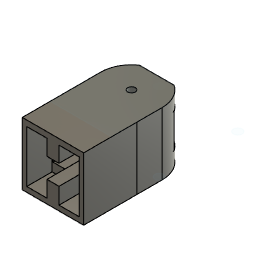
EndCap__FreeWheel (Autodesk Fusion 360 design; units mm, degrees)
Autodesk Fusion 360 part; units mm, degrees
(part 1 of 2)
sketch "Sketch1" plane through (0, 0, 0) normal (1, 0, 0) x (0, 0, -1)
  line L0 (0, 0) -> (-20, 0)
  line L1 (-20, 0) -> (-20, 20)
  line L2 (-20, 20) -> (0, 20)
  line L3 (0, 20) -> (0, 0)
  line L4 (-6.34, 6.34) -> (-13.66, 6.34)
  line L5 (-13.66, 6.34) -> (-13.66, 13.66)
  line L6 (-13.66, 13.66) -> (-6.34, 13.66)
  line L7 (-6.34, 13.66) -> (-6.34, 6.34)
  line L8 (-6.34, 6.34) -> (-13.66, 13.66) construction
  line L9 (-13.66, 6.34) -> (-6.34, 13.66) construction
  line L10 (-20, 20) -> (-20, 18.5)
  line L11 (-20, 18.5) -> (-18.5, 18.5)
  line L12 (-18.5, 18.5) -> (-1.5, 18.5)
  line L13 (-1.5, 18.5) -> (-1.5, 1.5)
  line L14 (-1.5, 1.5) -> (-18.5, 1.5)
  line L15 (-18.5, 1.5) -> (-18.5, 18.5)
  line L16 (-20, 0) -> (-20, 7.37)
  line L17 (-20, 7.37) -> (0, 7.37)
  line L18 (0, 7.37) -> (0, 12.63)
  line L19 (0, 12.63) -> (-20, 12.63)
  line L20 (-20, 12.63) -> (-20, 7.37)
  line L21 (-20, 0) -> (-12.63, 0)
  line L22 (-12.63, 0) -> (-7.37, 0)
  line L23 (-7.37, 0) -> (-7.37, 20.1614)
  line L24 (-7.37, 20.1614) -> (-12.63, 20.1614)
  line L25 (-12.63, 20.1614) -> (-12.63, 0)
  line L26 (-18.5, 18.5) -> (-1.5, 1.5)
  line L27 (-10, 10) -> (-9.4697, 10.5303)
  line L28 (-9.4697, 10.5303) -> (-17.4393, 18.5)
  line L29 (-9.4697, 10.5303) -> (1.8011, 10.5303) construction
  line L30 (-9.4697, 10.5303) -> (-1.5, 2.5607)
  line L31 (-10, 10) -> (-10.5303, 9.4697)
  line L32 (-10.5303, 9.4697) -> (-18.5, 17.4393)
  line L33 (-10.5303, 9.4697) -> (-2.5607, 1.5)
  line L34 (-10, 10) -> (-9.4697, 9.4697)
  line L35 (-9.4697, 9.4697) -> (-1.5, 17.4393)
  line L36 (-9.4697, 9.4697) -> (-17.4393, 1.5)
  line L37 (-10, 10) -> (-10.5303, 10.5303)
  line L38 (-10.5303, 10.5303) -> (-2.5607, 18.5)
  line L39 (-10.5303, 10.5303) -> (-18.5, 2.5607)
  line L40 (-10, 18.5) -> (-4.005, 18.5)
  line L41 (-4.005, 18.5) -> (-15.995, 18.5)
  line L42 (-15.995, 18.5) -> (-15.995, 17.0557)
  line L43 (-15.995, 17.0557) -> (-4.005, 17.0557)
  line L44 (-4.005, 17.0557) -> (-4.005, 18.5)
  line L45 (-15.995, 1.5) -> (-4.005, 1.5)
  line L46 (-4.005, 1.5) -> (-4.005, 2.9443)
  line L47 (-4.005, 2.9443) -> (-15.995, 2.9443)
  line L48 (-15.995, 2.9443) -> (-15.995, 1.5)
  line L49 (-18.5, 10) -> (-18.5, 4.005)
  line L50 (-18.5, 4.005) -> (-17.0557, 4.005)
  line L51 (-17.0557, 4.005) -> (-17.0557, 15.995)
  line L52 (-17.0557, 15.995) -> (-18.5, 15.995)
  line L53 (-18.5, 15.995) -> (-18.5, 4.005)
  line L54 (-1.5, 10) -> (-1.5, 4.005)
  line L55 (-1.5, 4.005) -> (-2.9443, 4.005)
  line L56 (-2.9443, 4.005) -> (-2.9443, 15.995)
  line L57 (-2.9443, 15.995) -> (-1.5, 15.995)
  line L58 (-1.5, 15.995) -> (-1.5, 4.005)
  point P0 (-10, 10)
  dimension "d1" = 20
  dimension "d2" = 20
  dimension "d3" = 7.32
  dimension "d4" = 7.32
  dimension "d5" = 1.5
  dimension "d6" = 1.5
  dimension "d7" = 17
  dimension "d8" = 17
  dimension "d9" = 7.37
  dimension "d10" = 5.26
  dimension "d11" = 7.37
  dimension "d12" = 5.26
  dimension "d13" = 0.75
  dimension "d14" = 135
  dimension "d15" = 45
  dimension "d16" = 0.75
  dimension "d17" = 0.75
  dimension "d18" = 0.75
  dimension "d19" = 5.995
  dimension "d20" = 11.99
  dimension "d21" = 11.99
  dimension "d22" = 5.995
  dimension "d23" = 11.99
  dimension "d24" = 5.995
  dimension "d25" = 11.99
  constraint horizontal L0
  constraint vertical L1
  constraint horizontal L2
  constraint vertical L3
  constraint coincident L0.start L3.end
  constraint perpendicular L4 L5
  constraint parallel L4 L6
  constraint parallel L5 L7
  constraint horizontal L4
  constraint coincident L8 P0
  constraint coincident L9 P0
  constraint perpendicular L2 L10
  constraint perpendicular L1 L11
  constraint horizontal L12
  constraint vertical L13
  constraint horizontal L14
  constraint vertical L15
  constraint perpendicular L0 L16
  constraint horizontal L17
  constraint vertical L18
  constraint horizontal L19
  constraint vertical L20
  constraint perpendicular L1 L21
  constraint horizontal L22
  constraint vertical L23
  constraint horizontal L24
  constraint vertical L25
  constraint coincident P0 L27.start
  constraint perpendicular L26 L27
  constraint horizontal L29
  constraint coincident L12 L28.end
  constraint coincident L13 L30.end
  constraint perpendicular L26 L31
  constraint coincident L15 L32.end
  constraint perpendicular L31 L32
  constraint coincident L14 L33.end
  constraint perpendicular L31 L33
  constraint perpendicular L31 L34
  constraint coincident L13 L35.end
  constraint perpendicular L30 L35
  constraint coincident L14 L36.end
  constraint perpendicular L34 L36
  constraint perpendicular L31 L37
  constraint coincident L12 L38.end
  constraint perpendicular L37 L38
  constraint coincident L15 L39.end
  constraint perpendicular L37 L39
  constraint midpoint L12 L40.start
  constraint perpendicular L23 L40
  constraint horizontal L41
  constraint vertical L42
  constraint horizontal L43
  constraint vertical L44
  constraint coincident L28 L42.end
  constraint horizontal L45
  constraint vertical L46
  constraint horizontal L47
  constraint vertical L48
  constraint coincident L33 L46.end
  constraint coincident L14 L45.start
  constraint vertical L49
  constraint midpoint L15 L49.start
  constraint horizontal L50
  constraint vertical L51
  constraint horizontal L52
  constraint vertical L53
  constraint coincident L32 L51.end
  constraint vertical L54
  constraint midpoint L13 L54.start
  constraint horizontal L55
  constraint vertical L56
  constraint horizontal L57
  constraint vertical L58
  constraint coincident L35 L56.end
  measures "d1" distance of L0.start L0.end
  measures "d2" distance of L0.start L2.end
  measures "d3" distance of L5.end L6.end
  measures "d4" distance of L4.end L5.end L0.start
  measures "d5" distance of L1.end L10.end
  measures "d6" distance of L10.end L11.end
  measures "d7" distance of L11.end L14.end
  measures "d8" distance of L11.end L12.end
  measures "d9" distance of L0.end L16.end
  measures "d10" distance of L16.end L19.end
  measures "d11" distance of L0.end L21.end
  measures "d12" distance of L21.end L22.end
  measures "d13" distance of P0 L27.end
  measures "d14" angle of L28 L29
  measures "d15" angle of L29 L30
  measures "d16" distance of P0 L31.end
  measures "d17" distance of P0 L34.end
  measures "d18" distance of P0 L37.end
  measures "d19" distance of L40.start L40.end
  measures "d20" distance of L40.end L41.end
  measures "d21" distance of L45.start L45.end
  measures "d22" distance of L49.start L49.end
  measures "d23" distance of L49.end L52.end
  measures "d24" distance of L54.start L54.end
  measures "d25" distance of L54.end L57.end
extrude "Extrude1" add sketch "Sketch1" along normal blind 10 contours L0 L3 L13 L14 L17 L23 L45 L54 L58 | L0 L1 L14 L15 L16 L17 L21 L25 L45 L49 L53 | L2 L3 L12 L13 L19 L23 L40 L41 L58 | L14 L33 L46 | L13 L30 L55 | L14 L36 L48 | L4 L14 L23 L26 L33 | L13 L35 L57 | L7 L13 L17 L26 L30 | L1 L11 L15 L19 L53 | L4 L5 L14 L15 L17 L25 L36 L39 | L4 L23 L26 | L4 L17 L23 L33 | L4 L17 L33 L36 | L1 L2 L10 L11 L12 L25 L41 | L6 L7 L12 L13 L19 L23 L35 L38 | L7 L17 L23 L30 | L7 L17 L26 | L7 L23 L30 L35 | L15 L39 L50 | L4 L17 L25 L36 | L4 L5 L17 L25 | L23 L26 L30 L35 | L17 L26 L33 L36 | L17 L33 L36 | L12 L38 L44 | L6 L7 L19 L23 | L7 L19 L23 L35 | L23 L30 L35 | L5 L15 L19 L26 L32 | L6 L12 L25 L26 L28 | L17 L25 L32 L33 L36 L39 | L5 L17 L25 L39 | L26 L31 L33 L34 L36 | L26 L27 L30 L34 L35 | L19 L23 L28 L30 L35 L38 | L6 L19 L23 L38 | L5 L19 L26 | L6 L25 L26 | L5 L25 L32 L39 | L25 L32 L39 | L26 L31 L32 L37 L39 | L26 L27 L28 L37 L38 | L6 L19 L28 L38 | L19 L28 L38 | L5 L19 L25 L32 | L6 L19 L25 L28 | L25 L26 L32 L39 | L19 L26 L28 L38 makes body 1
sketch "Sketch2" plane through (10, 0, 0) normal (1, 0, 0) x (0, 0, -1)
  line L0 (-6.3093, 12.63) -> (-2.9443, 15.995)
  line L1 (-2.9443, 15.995) -> (-1.5, 15.995)
  line L2 (-1.5, 15.995) -> (-1.5, 12.63)
  line L3 (-1.5, 12.63) -> (0, 12.63)
  line L4 (0, 12.63) -> (0, 20)
  line L5 (0, 20) -> (-7.37, 20)
  line L6 (-7.37, 20) -> (-7.37, 18.5)
  line L7 (-7.37, 18.5) -> (-4.005, 18.5)
  line L8 (-4.005, 18.5) -> (-4.005, 17.0557)
  line L9 (-4.005, 17.0557) -> (-7.37, 13.6907)
  line L10 (-7.37, 13.6907) -> (-7.37, 13.66)
  line L11 (-7.37, 13.66) -> (-12.63, 13.66)
  line L12 (-12.63, 13.66) -> (-12.63, 13.6907)
  line L13 (-12.63, 13.6907) -> (-17.4393, 18.5)
  line L14 (-17.4393, 18.5) -> (-12.63, 18.5)
  line L15 (-12.63, 18.5) -> (-12.63, 20)
  line L16 (-12.63, 20) -> (-20, 20)
  line L17 (-20, 20) -> (-20, 12.63)
  line L18 (-20, 12.63) -> (-18.5, 12.63)
  line L19 (-18.5, 12.63) -> (-18.5, 17.4393)
  line L20 (-18.5, 17.4393) -> (-13.6907, 12.63)
  line L21 (-13.6907, 12.63) -> (-13.66, 12.63)
  line L22 (-13.66, 12.63) -> (-13.66, 7.37)
  line L23 (-13.66, 7.37) -> (-13.6907, 7.37)
  line L24 (-13.6907, 7.37) -> (-17.0557, 4.005)
  line L25 (-17.0557, 4.005) -> (-18.5, 4.005)
  line L26 (-18.5, 4.005) -> (-18.5, 7.37)
  line L27 (-18.5, 7.37) -> (-20, 7.37)
  line L28 (-20, 7.37) -> (-20, 0)
  line L29 (-20, 0) -> (-12.63, 0)
  line L30 (-12.63, 0) -> (-12.63, 1.5)
  line L31 (-12.63, 1.5) -> (-15.995, 1.5)
  line L32 (-15.995, 1.5) -> (-15.995, 2.9443)
  line L33 (-15.995, 2.9443) -> (-12.63, 6.3093)
  line L34 (-12.63, 6.3093) -> (-12.63, 6.34)
  line L35 (-12.63, 6.34) -> (-7.37, 6.34)
  line L36 (-7.37, 6.34) -> (-7.37, 6.3093)
  line L37 (-7.37, 6.3093) -> (-4.005, 2.9443)
  line L38 (-4.005, 2.9443) -> (-4.005, 1.5)
  line L39 (-4.005, 1.5) -> (-7.37, 1.5)
  line L40 (-7.37, 1.5) -> (-7.37, 0)
  line L41 (-7.37, 0) -> (0, 0)
  line L42 (0, 0) -> (0, 7.37)
  line L43 (0, 7.37) -> (-1.5, 7.37)
  line L44 (-1.5, 7.37) -> (-1.5, 4.005)
  line L45 (-1.5, 4.005) -> (-2.9443, 4.005)
  line L46 (-2.9443, 4.005) -> (-6.3093, 7.37)
  line L47 (-6.3093, 7.37) -> (-6.34, 7.37)
  line L48 (-6.34, 7.37) -> (-6.34, 12.63)
  line L49 (-6.34, 12.63) -> (-6.3093, 12.63)
  line L50 (-6.34, 10) -> (-10, 10)
  circle A0 centre (-10, 10) radius 2.095
  dimension "d28" = 4.19
  constraint midpoint L48 L50.start
  constraint perpendicular L48 L50
  constraint coincident L50.end A0.centre
  measures "d28" diameter of A0
extrude "Extrude2" cut sketch "Sketch2" against normal blind 10 contours A0 bodies 1
fillet "Fillet1" radius 1.5 4 edges at (5, 0, 0) (5, 0, 20) (5, 20, 0) (5, 20, 20) on bodies 1
sketch "Sketch3" plane through (10, 0, 0) normal (1, 0, 0) x (0, 0, -1)
  arc A0 (-18.5, 20) -> (-20, 18.5) centre (-18.5, 18.5) ccw
  line L0 (-20, 18.5) -> (-20, 12.63)
  line L1 (-20, 12.63) -> (-18.5, 12.63)
  line L2 (-18.5, 12.63) -> (-18.5, 17.4393)
  line L3 (-18.5, 17.4393) -> (-13.6907, 12.63)
  line L4 (-13.6907, 12.63) -> (-13.66, 12.63)
  line L5 (-13.66, 12.63) -> (-13.66, 7.37)
  line L6 (-13.66, 7.37) -> (-13.6907, 7.37)
  line L7 (-13.6907, 7.37) -> (-17.0557, 4.005)
  line L8 (-17.0557, 4.005) -> (-18.5, 4.005)
  line L9 (-18.5, 4.005) -> (-18.5, 7.37)
  line L10 (-18.5, 7.37) -> (-20, 7.37)
  line L11 (-20, 7.37) -> (-20, 1.5)
  arc A1 (-20, 1.5) -> (-18.5, 0) centre (-18.5, 1.5) ccw
  line L12 (-18.5, 0) -> (-12.63, 0)
  line L13 (-12.63, 0) -> (-12.63, 1.5)
  line L14 (-12.63, 1.5) -> (-15.995, 1.5)
  line L15 (-15.995, 1.5) -> (-15.995, 2.9443)
  line L16 (-15.995, 2.9443) -> (-12.63, 6.3093)
  line L17 (-12.63, 6.3093) -> (-12.63, 6.34)
  line L18 (-12.63, 6.34) -> (-7.37, 6.34)
  line L19 (-7.37, 6.34) -> (-7.37, 6.3093)
  line L20 (-7.37, 6.3093) -> (-4.005, 2.9443)
  line L21 (-4.005, 2.9443) -> (-4.005, 1.5)
  line L22 (-4.005, 1.5) -> (-7.37, 1.5)
  line L23 (-7.37, 1.5) -> (-7.37, 0)
  line L24 (-7.37, 0) -> (-1.5, 0)
  arc A2 (-1.5, 0) -> (0, 1.5) centre (-1.5, 1.5) ccw
  line L25 (0, 1.5) -> (0, 7.37)
  line L26 (0, 7.37) -> (-1.5, 7.37)
  line L27 (-1.5, 7.37) -> (-1.5, 4.005)
  line L28 (-1.5, 4.005) -> (-2.9443, 4.005)
  line L29 (-2.9443, 4.005) -> (-6.3093, 7.37)
  line L30 (-6.3093, 7.37) -> (-6.34, 7.37)
  line L31 (-6.34, 7.37) -> (-6.34, 12.63)
  line L32 (-6.34, 12.63) -> (-6.3093, 12.63)
  line L33 (-6.3093, 12.63) -> (-2.9443, 15.995)
  line L34 (-2.9443, 15.995) -> (-1.5, 15.995)
  line L35 (-1.5, 15.995) -> (-1.5, 12.63)
  line L36 (-1.5, 12.63) -> (0, 12.63)
  line L37 (0, 12.63) -> (0, 18.5)
  arc A3 (0, 18.5) -> (-1.5, 20) centre (-1.5, 18.5) ccw
  line L38 (-1.5, 20) -> (-7.37, 20)
  line L39 (-7.37, 20) -> (-7.37, 18.5)
  line L40 (-7.37, 18.5) -> (-4.005, 18.5)
  line L41 (-4.005, 18.5) -> (-4.005, 17.0557)
  line L42 (-4.005, 17.0557) -> (-7.37, 13.6907)
  line L43 (-7.37, 13.6907) -> (-7.37, 13.66)
  line L44 (-7.37, 13.66) -> (-12.63, 13.66)
  line L45 (-12.63, 13.66) -> (-12.63, 13.6907)
  line L46 (-12.63, 13.6907) -> (-17.4393, 18.5)
  line L47 (-17.4393, 18.5) -> (-12.63, 18.5)
  line L48 (-12.63, 18.5) -> (-12.63, 20)
  line L49 (-12.63, 20) -> (-18.5, 20)
  circle A4 centre (-10, 10) radius 2.095
  line L50 (-4.005, 17.0557) -> (-15.995, 17.0557)
  line L51 (-17.0557, 4.005) -> (-17.0557, 15.995)
  line L52 (-17.0557, 15.995) -> (-18.5, 15.995)
  line L53 (-15.995, 17.0557) -> (-15.995, 18.5)
  constraint coincident L41.end L42.start
  constraint coincident L46 L50.end
  constraint perpendicular L41 L50
  constraint coincident L7.end L8.start
  constraint coincident L3 L51.end
  constraint perpendicular L8 L51
  constraint coincident L2 L52.end
  constraint perpendicular L2 L52
  constraint coincident L47 L53.end
  constraint perpendicular L47 L53
extrude "Extrude3" add sketch "Sketch3" against normal blind 10 contours L46 L47 L53 | L2 L3 L52 bodies 1
sketch "Sketch4" plane through (0, 0, 0) normal (0, 1, 0) x (1, 0, 0)
  line L0 (25, 0) -> (67, 0)
  line L1 (67, 0) -> (67, -42)
  line L2 (67, -42) -> (25, -42)
  line L3 (25, -42) -> (25, 0)
  line L4 (46, 0) -> (46, -21)
  line L5 (61.5, -36.5) -> (61.5, -5.5)
  line L6 (61.5, -5.5) -> (30.5, -36.5) construction
  line L7 (30.5, -5.5) -> (61.5, -36.5) construction
  circle A0 centre (30.5, -5.5) radius 1.75
  circle A1 centre (61.5, -5.5) radius 1.75
  circle A2 centre (30.5, -36.5) radius 1.75
  circle A3 centre (61.5, -36.5) radius 1.75
  point P0 (46, -21)
  dimension "d34" = 42
  dimension "d35" = 42
  dimension "d36" = 21
  dimension "d37" = 31
  dimension "d38" = 31
  dimension "d39" = 3.5
  dimension "d40" = 3.5
  dimension "d41" = 3.5
  dimension "d42" = 3.5
  constraint horizontal L0
  constraint vertical L1
  constraint horizontal L2
  constraint vertical L3
  constraint midpoint L0 L4.start
  constraint perpendicular L0 L4
  constraint coincident L6 P0
  constraint coincident L7 P0
  constraint coincident P0 L4.end
  constraint coincident L7.start A0.centre
  constraint coincident L5.end L6.start
  constraint coincident L6.end A2.centre
  constraint coincident L5.start L7.end
  measures "d34" distance of L0.start L2.end
  measures "d35" distance of L0.start L0.end
  measures "d36" distance of L4.start P0
  measures "d37" distance of L6.end L5.start
  measures "d38" distance of L7.start L6.end
  measures "d39" diameter of A0
  measures "d40" diameter of A1
  measures "d41" diameter of A2
  measures "d42" diameter of A3
extrude "Extrude4" add sketch "Sketch4" along normal blind 5 separate body makes body 2
sketch "Sketch5" plane through (25, 0, 0) normal (-1, 0, 0) x (0, 0, 1)
  line L0 (0, 0) -> (42, 0)
  line L1 (42, 0) -> (42, 5)
  line L2 (42, 5) -> (0, 5)
  line L3 (0, 5) -> (0, 0)
  line L4 (42, 0) -> (31, 0)
  line L5 (31, 0) -> (11, 0)
  line L6 (11, 0) -> (11, 20)
  line L7 (11, 20) -> (31, 20)
  line L8 (31, 20) -> (31, 0)
  line L9 (31, 0) -> (31, 1.5)
  line L10 (31, 1.5) -> (29.5, 1.5)
  line L11 (29.5, 1.5) -> (12.5, 1.5)
  line L12 (12.5, 1.5) -> (12.5, 18.5)
  line L13 (12.5, 18.5) -> (29.5, 18.5)
  line L14 (29.5, 18.5) -> (29.5, 1.5)
  line L15 (21, 1.5) -> (23.5, 1.5)
  line L16 (23.5, 1.5) -> (18.5, 1.5)
  line L17 (18.5, 1.5) -> (18.5, 0)
  line L18 (18.5, 0) -> (23.5, 0)
  line L19 (23.5, 0) -> (23.5, 1.5)
  line L20 (11, 10) -> (21, 10)
  line L21 (21, 10) -> (21.5303, 10.5303)
  line L22 (21, 10) -> (21.5303, 9.4697)
  line L23 (21, 10) -> (21.75, 10) construction
  line L24 (21.5303, 10.5303) -> (13.5607, 18.5)
  line L25 (21.5303, 10.5303) -> (29.5, 2.5607)
  line L26 (21.5303, 9.4697) -> (29.5, 17.4393)
  line L27 (21.5303, 9.4697) -> (13.5607, 1.5)
  line L28 (21, 10) -> (20.4697, 9.4697)
  line L29 (20.4697, 9.4697) -> (12.5, 17.4393)
  line L30 (21, 8.9393) -> (28.4393, 1.5)
  line L31 (21, 10) -> (20.4697, 10.5303)
  line L32 (20.4697, 10.5303) -> (12.5, 2.5607)
  line L33 (20.4697, 10.5303) -> (28.4393, 18.5)
  line L34 (24.66, 6.34) -> (17.34, 6.34)
  line L35 (17.34, 6.34) -> (17.34, 13.66)
  line L36 (17.34, 13.66) -> (24.66, 13.66)
  line L37 (24.66, 13.66) -> (24.66, 6.34)
  line L38 (24.66, 6.34) -> (17.34, 13.66) construction
  line L39 (17.34, 6.34) -> (24.66, 13.66) construction
  line L40 (21, 1.5) -> (26.75, 1.5)
  line L41 (26.75, 1.5) -> (15.25, 1.5)
  line L42 (15.25, 1.5) -> (15.25, 3.1893)
  line L43 (15.25, 3.1893) -> (26.75, 3.1893)
  line L44 (26.75, 3.1893) -> (26.75, 1.5)
  line L45 (15.25, 18.5) -> (26.75, 18.5)
  line L46 (26.75, 18.5) -> (26.75, 16.8107)
  line L47 (26.75, 16.8107) -> (15.25, 16.8107)
  line L48 (15.25, 16.8107) -> (15.25, 18.5)
  point P0 (21, 10)
  dimension "d45" = 20
  dimension "d46" = 20
  dimension "d47" = 1.5
  dimension "d48" = 1.5
  dimension "d49" = 2.5
  dimension "d50" = 5
  dimension "d51" = 1.5
  dimension "d53" = 0.75
  dimension "d54" = 45
  dimension "d55" = 0.75
  dimension "d56" = 0.75
  dimension "d57" = 7.32
  dimension "d58" = 7.32
  dimension "d59" = 5.75
  dimension "d60" = 11.5
  constraint coincident L0.end L1.start
  constraint coincident L0 L4.end
  constraint horizontal L5
  constraint vertical L6
  constraint horizontal L7
  constraint vertical L8
  constraint perpendicular L4 L9
  constraint perpendicular L8 L10
  constraint horizontal L11
  constraint vertical L12
  constraint horizontal L13
  constraint vertical L14
  constraint midpoint L11 L15.start
  constraint parallel L11 L15
  constraint horizontal L16
  constraint vertical L17
  constraint horizontal L18
  constraint vertical L19
  constraint midpoint L6 L20.start
  constraint perpendicular L14 L20
  constraint horizontal L23
  constraint perpendicular L21 L22
  constraint coincident L13 L24.end
  constraint perpendicular L21 L24
  constraint coincident L14 L25.end
  constraint perpendicular L21 L25
  constraint coincident L14 L26.end
  constraint perpendicular L25 L26
  constraint coincident L11 L27.end
  constraint perpendicular L22 L27
  constraint perpendicular L22 L28
  constraint coincident L12 L29.end
  constraint perpendicular L27 L29
  constraint coincident L27 L30.start
  constraint coincident L11 L30.end
  constraint perpendicular L27 L30
  constraint perpendicular L28 L31
  constraint coincident L12 L32.end
  constraint perpendicular L31 L32
  constraint coincident L13 L33.end
  constraint perpendicular L31 L33
  constraint perpendicular L34 L35
  constraint parallel L34 L36
  constraint parallel L35 L37
  constraint horizontal L34
  constraint coincident L38 P0
  constraint coincident L39 P0
  constraint coincident P0 L20.end
  constraint parallel L11 L40
  constraint horizontal L41
  constraint vertical L42
  constraint horizontal L43
  constraint vertical L44
  constraint coincident L27 L42.end
  constraint horizontal L45
  constraint vertical L46
  constraint horizontal L47
  constraint vertical L48
  constraint coincident L33 L46.end
  constraint coincident L13 L45.start
  measures "d45" distance of L4.end L7.end
  measures "d46" distance of L4.end L5.end
  measures "d47" distance of L4.end L9.end
  measures "d48" distance of L9.end L10.end
  measures "d49" distance of L15.start L15.end
  measures "d50" distance of L15.end L16.end
  measures "d51" distance of L15.end L18.end
  measures "d53" distance of P0 L21.end
  measures "d54" angle of L22 L23
  measures "d55" distance of P0 L22.end
  measures "d56" distance of P0 L31.end
  measures "d57" distance of L34.end L35.end
  measures "d58" distance of L35.end L36.end
  measures "d59" distance of L15.start L40.end
  measures "d60" distance of L40.end L41.end
extrude "Extrude5" add sketch "Sketch5" along normal blind 5 contours L11 L15 L16 L40 L41 L42 L43 L44 | L2 L27 L30 L43 | L2 L27 L30 L34 | L13 L45 L46 L47 L48 | L24 L33 L36 L47 bodies 2 makes body 3 at (23.3333, 18.5, 19.0833)
sketch "Sketch6" plane through (25, 0, 0) normal (-1, 0, 0) x (0, 0, 1)
  line L0 (15.25, 3.1893) -> (17.0607, 5)
  line L1 (17.0607, 5) -> (0, 5)
  line L2 (0, 5) -> (0, 0)
  line L3 (0, 0) -> (42, 0)
  line L4 (42, 0) -> (42, 5)
  line L5 (42, 5) -> (24.9393, 5)
  line L6 (24.9393, 5) -> (26.75, 3.1893)
  line L7 (26.75, 3.1893) -> (26.75, 1.5)
  line L8 (26.75, 1.5) -> (15.25, 1.5)
  line L9 (15.25, 1.5) -> (15.25, 3.1893)
  line L10 (42, 0) -> (31, 0)
  line L11 (31, 0) -> (11, 0)
  line L12 (11, 0) -> (11, 20)
  line L13 (11, 20) -> (31, 20)
  line L14 (31, 20) -> (31, 0)
  line L15 (24.9393, 5) -> (17.0603, 5)
  line L16 (17.0603, 5) -> (17.0603, 18.4957)
  line L17 (17.0603, 18.4957) -> (24.9393, 18.4957)
  line L18 (24.9393, 18.4957) -> (24.9393, 5)
  dimension "d63" = 20
  dimension "d64" = 20
  dimension "d65" = 7.879
  constraint coincident L3.end L4.start
  constraint coincident L3 L10.end
  constraint horizontal L11
  constraint vertical L12
  constraint horizontal L13
  constraint vertical L14
  constraint horizontal L15
  constraint vertical L16
  constraint horizontal L17
  constraint vertical L18
  constraint coincident L5.end L6.start
  measures "d63" distance of L10.end L11.end
  measures "d64" distance of L10.end L13.end
  measures "d65" distance of L5.end L15.end
extrude "Extrude6" add sketch "Sketch6" against normal blind 9 contours L15 L16 L17 L18 bodies 2 3
sketch "Sketch7" plane through (25, 0, 0) normal (-1, 0, 0) x (0, 0, 1)
  line L0 (18.4007, 13.66) -> (17.0603, 15.0003)
  line L1 (17.0603, 15.0003) -> (17.0603, 5)
  line L2 (17.0603, 5) -> (0, 5)
  line L3 (0, 5) -> (0, 0)
  line L4 (0, 0) -> (42, 0)
  line L5 (42, 0) -> (42, 5)
  line L6 (42, 5) -> (24.9393, 5)
  line L7 (24.9393, 5) -> (26.75, 3.1893)
  line L8 (26.75, 3.1893) -> (26.75, 1.5)
  line L9 (26.75, 1.5) -> (15.25, 1.5)
  line L10 (15.25, 1.5) -> (15.25, 3.1893)
  line L11 (15.25, 3.1893) -> (18.4007, 6.34)
  line L12 (18.4007, 6.34) -> (23.5993, 6.34)
  line L13 (23.5993, 6.34) -> (24.9393, 5)
  line L14 (24.9393, 5) -> (24.9393, 15)
  line L15 (24.9393, 15) -> (23.5993, 13.66)
  line L16 (23.5993, 13.66) -> (18.4007, 13.66)
  line L17 (21, 0) -> (23.5, 0)
  line L18 (23.5, 0) -> (18.5, 0)
  line L19 (18.5, 0) -> (18.5, 1.5)
  line L20 (18.5, 1.5) -> (23.5, 1.5)
  line L21 (23.5, 1.5) -> (23.5, 0)
  dimension "d68" = 2.5
  dimension "d69" = 5
  dimension "d70" = 1.5
  constraint midpoint L4 L17.start
  constraint parallel L4 L17
  constraint horizontal L18
  constraint vertical L19
  constraint horizontal L20
  constraint vertical L21
  measures "d68" distance of L17.start L17.end
  measures "d69" distance of L17.end L18.end
  measures "d70" distance of L17.end L20.end
extrude "Extrude7" add sketch "Sketch7" along normal blind 5 contours L4 L9 L17 L18 L19 L20 L21 bodies 2
sketch "Sketch8" plane through (34, 0, 0) normal (1, 0, 0) x (0, 0, -1)
  line L0 (-17.0603, 18.4957) -> (-24.9393, 18.4957)
  line L1 (-24.9393, 18.4957) -> (-24.9393, 5)
  line L2 (-24.9393, 5) -> (-17.0603, 5)
  line L3 (-17.0603, 5) -> (-17.0603, 18.4957)
  line L4 (-17.0603, 5) -> (-20.9998, 5)
  line L5 (-20.9998, 5) -> (-20.9998, 10)
  circle A0 centre (-20.9998, 10) radius 2.25
  dimension "d73" = 4.5
  constraint coincident L2.end L3.start
  constraint midpoint L2 L4.end
  constraint perpendicular L4 L5
  constraint coincident L5.end A0.centre
  measures "d73" diameter of A0
extrude "Extrude8" cut sketch "Sketch8" against normal blind 19 contours A0 bodies 2
sketch "Sketch9" plane through (20, 0, 0) normal (-1, 0, 0) x (0, 0, 1)
  line L0 (23.5993, 6.34) -> (18.4007, 6.34)
  line L1 (18.4007, 6.34) -> (15.25, 3.1893)
  line L2 (15.25, 3.1893) -> (15.25, 1.5)
  line L3 (15.25, 1.5) -> (18.5, 1.5)
  line L4 (18.5, 1.5) -> (18.5, 0)
  line L5 (18.5, 0) -> (23.5, 0)
  line L6 (23.5, 0) -> (23.5, 1.5)
  line L7 (23.5, 1.5) -> (26.75, 1.5)
  line L8 (26.75, 1.5) -> (26.75, 3.1893)
  line L9 (26.75, 3.1893) -> (23.5993, 6.34)
  line L10 (18.5, 1.5) -> (16.0303, 3.9697)
  line L11 (23.5, 1.5) -> (25.9697, 3.9697)
  constraint coincident L3.end L4.start
  constraint coincident L1 L10.end
  constraint perpendicular L1 L10
  constraint coincident L6.end L7.start
  constraint coincident L9 L11.end
  constraint perpendicular L9 L11
extrude "Extrude9" cut sketch "Sketch9" against normal blind 5 contours L7 L8 L9 L11 | L1 L2 L3 L10 bodies 2
sketch "Sketch10" plane through (0, 0, 0) normal (0, -1, 0) x (1, 0, 0)
  circle A0 centre (30.5, 5.5) radius 1.75
  circle A1 centre (30.5, 36.5) radius 1.75
  circle A2 centre (61.5, 5.5) radius 1.75
  circle A3 centre (61.5, 36.5) radius 1.75
  line L0 (67, 42) -> (25, 42)
  line L1 (25, 42) -> (25, 23.5)
  line L2 (25, 23.5) -> (20, 23.5)
  line L3 (20, 23.5) -> (20, 18.5)
  line L4 (20, 18.5) -> (25, 18.5)
  line L5 (25, 18.5) -> (25, 0)
  line L6 (25, 0) -> (67, 0)
  line L7 (67, 0) -> (67, 42)
  line L8 (46, 0) -> (46, 20)
  circle A4 centre (46, 20) radius 8.625
  dimension "d78" = 17.25
  constraint midpoint L6 L8.start
  constraint perpendicular L6 L8
  constraint coincident L8.end A4.centre
  measures "d78" diameter of A4
sketch "Sketch11" plane through (0, 0, 0) normal (0, -1, 0) x (1, 0, 0)
  circle A0 centre (30.5, 5.5) radius 1.75
  circle A1 centre (30.5, 36.5) radius 1.75
  circle A2 centre (61.5, 5.5) radius 1.75
  circle A3 centre (61.5, 36.5) radius 1.75
  line L0 (67, 42) -> (25, 42)
  line L1 (25, 42) -> (25, 23.5)
  line L2 (25, 23.5) -> (20, 23.5)
  line L3 (20, 23.5) -> (20, 18.5)
  line L4 (20, 18.5) -> (25, 18.5)
  line L5 (25, 18.5) -> (25, 0)
  line L6 (25, 0) -> (67, 0)
  line L7 (67, 0) -> (67, 42)
  circle A4 centre (46, 20) radius 12
  dimension "d81" = 24
  measures "d81" diameter of A4
extrude "Extrude12" add 2 faces at (20, 4.7267, 21.8333) (20, 16.8867, 21.8664) along direction (-1, 0, 0) blind 5 on bodies 2 bodies 2
sketch "Sketch12" plane through (0, 18.5, 0) normal (0, 1, 0) x (-1, 0, 0)
  line L0 (-25, 26.75) -> (-25, 15.25)
  line L1 (-25, 15.25) -> (-15, 15.25)
  line L2 (-15, 15.25) -> (-15, 26.75)
  line L3 (-15, 26.75) -> (-25, 26.75)
  line L4 (-15, 21) -> (-20, 21)
  circle A0 centre (-20, 21) radius 1.25
  dimension "d86" = 2.5
  constraint midpoint L2 L4.start
  constraint perpendicular L0 L4
  constraint coincident L4.end A0.centre
  measures "d86" diameter of A0
extrude "Extrude13" cut sketch "Sketch12" against normal blind 21 contours A0 bodies 2
sketch "Sketch13" plane through (0, 0, 0) normal (0, -1, 0) x (1, 0, 0)
  circle A0 centre (20, 21) radius 1.25
  circle A1 centre (30.5, 5.5) radius 1.75
  circle A2 centre (30.5, 36.5) radius 1.75
  circle A3 centre (61.5, 5.5) radius 1.75
  circle A4 centre (61.5, 36.5) radius 1.75
  line L0 (67, 42) -> (25, 42)
  line L1 (25, 42) -> (25, 23.5)
  line L2 (25, 23.5) -> (15, 23.5)
  line L3 (15, 23.5) -> (15, 18.5)
  line L4 (15, 18.5) -> (25, 18.5)
  line L5 (25, 18.5) -> (25, 0)
  line L6 (25, 0) -> (67, 0)
  line L7 (67, 0) -> (67, 42)
  line L8 (46, 42) -> (46, 21)
  circle A5 centre (46, 21) radius 8.625
  dimension "d89" = 17.25
  constraint midpoint L0 L8.start
  constraint perpendicular L0 L8
  constraint coincident L8.end A5.centre
  measures "d89" diameter of A5
extrude "Extrude14" cut sketch "Sketch13" against normal blind 15 contours A5 bodies 2
sketch "Sketch14" plane through (0, 0, 0) normal (0, -1, 0) x (1, 0, 0)
  circle A0 centre (46, 21) radius 8.625
  circle A1 centre (20, 21) radius 1.25
  circle A2 centre (30.5, 5.5) radius 1.75
  circle A3 centre (30.5, 36.5) radius 1.75
  circle A4 centre (61.5, 5.5) radius 1.75
  circle A5 centre (61.5, 36.5) radius 1.75
  line L0 (67, 42) -> (25, 42)
  line L1 (25, 42) -> (25, 23.5)
  line L2 (25, 23.5) -> (15, 23.5)
  line L3 (15, 23.5) -> (15, 18.5)
  line L4 (15, 18.5) -> (25, 18.5)
  line L5 (25, 18.5) -> (25, 0)
  line L6 (25, 0) -> (67, 0)
  line L7 (67, 0) -> (67, 42)
  line L8 (67, 21) -> (46, 21)
  circle A6 centre (46, 21) radius 12
  dimension "d92" = 24
  constraint midpoint L7 L8.start
  constraint coincident A0.centre L8.end
  constraint concentric A0 A6
  measures "d92" diameter of A6
extrude "Extrude15" cut sketch "Sketch14" against normal blind 3 contours A6 bodies 2
extrude "Extrude16" cut 1 faces at (20.0311, 18.5, 16.7512) along direction (0, -1, 0) blind 1 on bodies 2 bodies 2
extrude "Extrude17" cut 1 faces at (28, 18.4957, 19.6867) along direction (0, -1, 0) blind 0.996 on bodies 2 bodies 2
sketch "Sketch15" plane through (0, -4.9697, 4.9697) normal (0, -0.707107, 0.707107) x (1, 0, 0)
sketch "Sketch16" plane through (15, 0, 0) normal (-1, 0, 0) x (0, 0, 1)
  line L0 (26.75, 17.5) -> (15.25, 17.5)
  line L1 (15.25, 17.5) -> (15.25, 16.8107)
  line L2 (15.25, 16.8107) -> (18.4007, 13.66)
  line L3 (18.4007, 13.66) -> (23.5993, 13.66)
  line L4 (23.5993, 13.66) -> (26.75, 16.8107)
  line L5 (26.75, 16.8107) -> (26.75, 17.5)
  line L6 (15.25, 17.5) -> (26.75, 17.5)
  line L7 (26.75, 17.5) -> (26.75, 13.66)
  line L8 (26.75, 13.66) -> (15.25, 13.66)
  line L9 (15.25, 13.66) -> (15.25, 17.5)
  dimension "d99" = 11.5
  constraint horizontal L6
  constraint vertical L7
  constraint horizontal L8
  constraint vertical L9
  constraint coincident L0.end L1.start
  measures "d99" distance of L0.end L0.start
extrude "Extrude18" add sketch "Sketch16" against normal blind 10 contours L4 L7 L8 | L2 L8 L9 bodies 2
extrude "Extrude19" cut 1 faces at (20.0311, 13.66, 16.7512) along direction (0, 1, 0) blind 0.5 on bodies 2 bodies 2
sketch "Sketch17" plane through (15, 0, 0) normal (-1, 0, 0) x (0, 0, 1)
  line L0 (15.25, 14.16) -> (26.75, 14.16)
  line L1 (26.75, 14.16) -> (26.75, 17.5)
  line L2 (26.75, 17.5) -> (15.25, 17.5)
  line L3 (15.25, 17.5) -> (15.25, 14.16)
  line L4 (21, 14.16) -> (23.505, 14.16)
  line L5 (23.505, 14.16) -> (18.405, 14.16)
  line L6 (18.405, 14.16) -> (15.25, 17.315)
  line L7 (18.405, 14.16) -> (22.8668, 14.16) construction
  line L8 (23.505, 14.16) -> (26.75, 17.405)
  dimension "d104" = 2.505
  dimension "d105" = 5.1
  dimension "d106" = 135
  constraint midpoint L0 L4.start
  constraint parallel L0 L4
  constraint parallel L0 L5
  constraint horizontal L7
  constraint coincident L3 L6.end
  constraint coincident L1 L8.end
  constraint perpendicular L6 L8
  measures "d104" distance of L4.start L4.end
  measures "d105" distance of L4.end L5.end
  measures "d106" angle of L6 L7
extrude "Extrude20" cut sketch "Sketch17" against normal blind 10 contours L0 L3 L6 | L0 L1 L8 bodies 2
sketch "Sketch18" plane through (0, 5, 0) normal (0, 1, 0) x (-1, 0, 0)
  circle A0 centre (-61.5, 36.5) radius 1.75
  circle A1 centre (-61.5, 5.5) radius 1.75
  circle A2 centre (-30.5, 5.5) radius 1.75
extrude "Extrude21" add 1 faces at (31, 12.2199, 24.9393) along direction (0, 0, 1) blind 1.811 on bodies 2 bodies 2
extrude "Extrude22" add 1 faces at (31, 12.6681, 17.0605) along direction (0, 0, -1) blind 1.81 on bodies 2 bodies 2
sketch "Sketch19" plane through (0, 5, 0) normal (0, 1, 0) x (-1, 0, 0)
  line L0 (-45, 0) -> (-39.25, 0)
  line L1 (-39.25, 0) -> (-50.75, 0)
  line L2 (-50.75, 0) -> (-50.75, 9)
  line L3 (-50.75, 9) -> (-39.25, 9)
  line L4 (-39.25, 9) -> (-39.25, 0)
  line L5 (-67, 42) -> (-67, 21)
  line L6 (-67, 21) -> (-67, 26.75)
  line L7 (-67, 26.75) -> (-58, 26.75)
  line L8 (-58, 26.75) -> (-58, 15.25)
  line L9 (-58, 15.25) -> (-67, 15.25)
  line L10 (-67, 15.25) -> (-67, 26.75)
  line L11 (-67, 42) -> (-46, 42)
  line L12 (-46, 42) -> (-40.25, 42)
  line L13 (-40.25, 42) -> (-51.75, 42)
  line L14 (-51.75, 42) -> (-51.75, 33)
  line L15 (-51.75, 33) -> (-40.25, 33)
  line L16 (-40.25, 33) -> (-40.25, 42)
  line L17 (-45, 0) -> (-45, 4.5)
  line L18 (-67, 21) -> (-62.5, 21)
  line L19 (-46, 42) -> (-46, 37.5)
  circle A0 centre (-46, 37.5) radius 1
  circle A1 centre (-62.5, 21) radius 1
  circle A2 centre (-45, 4.5) radius 1
  dimension "d113" = 5.75
  dimension "d114" = 11.5
  dimension "d115" = 9
  dimension "d116" = 5.75
  dimension "d117" = 9
  dimension "d118" = 11.5
  dimension "d119" = 5.75
  dimension "d120" = 11.5
  dimension "d121" = 9
  dimension "d122" = 4.5
  dimension "d123" = 4.5
  dimension "d124" = 4.5
  dimension "d125" = 2
  dimension "d126" = 2
  dimension "d127" = 2
  constraint horizontal L0
  constraint horizontal L1
  constraint vertical L2
  constraint horizontal L3
  constraint vertical L4
  constraint vertical L5
  constraint parallel L5 L6
  constraint horizontal L7
  constraint vertical L8
  constraint horizontal L9
  constraint vertical L10
  constraint perpendicular L5 L11
  constraint perpendicular L5 L12
  constraint horizontal L13
  constraint vertical L14
  constraint horizontal L15
  constraint vertical L16
  constraint perpendicular L3 L17
  constraint perpendicular L5 L18
  constraint perpendicular L12 L19
  constraint coincident L19.end A0.centre
  constraint coincident L18.end A1.centre
  constraint coincident L17.end A2.centre
  measures "d113" distance of L0.start L0.end
  measures "d114" distance of L0.end L1.end
  measures "d115" distance of L0.end L3.end
  measures "d116" distance of L5.end L6.end
  measures "d117" distance of L6.end L7.end
  measures "d118" distance of L6.end L9.end
  measures "d119" distance of L11.end L12.end
  measures "d120" distance of L12.end L13.end
  measures "d121" distance of L12.end L15.end
  measures "d122" distance of L0.start L17.end
  measures "d123" distance of L5.end L18.end
  measures "d124" distance of L11.end L19.end
  measures "d125" diameter of A0
  measures "d126" diameter of A1
  measures "d127" diameter of A2
extrude "Extrude23" add sketch "Sketch19" along normal blind 12.5 bodies 2
sketch "Sketch20" plane through (0, 17.4997, 0) normal (0, 1, 0) x (-1, 0, 0)
  line L0 (-25, 15.2503) -> (-25, 26.75)
  line L1 (-25, 26.75) -> (-25, 26.7503)
  line L2 (-25, 26.7503) -> (-34, 26.7503)
  line L3 (-34, 26.7503) -> (-34, 15.2503)
  line L4 (-34, 15.2503) -> (-25, 15.2503)
  line L5 (-25, 21.0002) -> (-29.5, 21.0002)
  circle A0 centre (-29.5, 21.0002) radius 1
  dimension "d130" = 4.5
  dimension "d131" = 2
  constraint midpoint L0 L5.start
  constraint perpendicular L0 L5
  constraint coincident L5.end A0.centre
  measures "d130" distance of L5.start L5.end
  measures "d131" diameter of A0
sketch "Sketch21" plane through (0, 5, 0) normal (0, 1, 0) x (-1, 0, 0)
sketch "Sketch22" plane through (0, 0, 0) normal (0, -1, 0) x (1, 0, 0)
  circle A0 centre (46, 21) radius 12
  circle A1 centre (20, 21) radius 1.25
  circle A2 centre (30.5, 5.5) radius 1.75
  circle A3 centre (30.5, 36.5) radius 1.75
  circle A4 centre (61.5, 5.5) radius 1.75
  circle A5 centre (61.5, 36.5) radius 1.75
  line L0 (67, 42) -> (25, 42)
  line L1 (25, 42) -> (25, 23.5)
  line L2 (25, 23.5) -> (15, 23.5)
  line L3 (15, 23.5) -> (15, 18.5)
  line L4 (15, 18.5) -> (25, 18.5)
  line L5 (25, 18.5) -> (25, 0)
  line L6 (25, 0) -> (67, 0)
  line L7 (67, 0) -> (67, 42)
  circle A6 centre (45, 4) radius 2.8284
  circle A7 centre (62.7598, 21) radius 1.8542
  circle A8 centre (46, 38) radius 2
extrude "Extrude25" add sketch "Sketch22" against normal blind 12.5 contours A6 | A7 | A8 bodies 2
extrude "Extrude26" cut 1 faces at (62.4751, 17.5, 16.8343) along direction (0, -1, 0) blind 12.5 on bodies 2 bodies 2
extrude "Extrude27" cut 1 faces at (61.7547, 12.5, 21.0497) along direction (0, -1, 0) blind 7.5 on bodies 2 bodies 2
fillet "Fillet2" radius 3 3 edges at (67, 2.5, 0) (67, 2.5, 42) (25, 2.5, 0) on bodies 2
fillet "Fillet3" radius 3 1 edges at (25, 2.5, 42) on bodies 2
sketch "Sketch23" plane through (0, 0, 15.2503) normal (0, 0, -1) x (-1, 0, 0)
  line L0 (-25, 17.4997) -> (-34, 17.4997)
  line L1 (-34, 17.4997) -> (-34, 5)
  line L2 (-34, 5) -> (-25, 5)
  line L3 (-25, 5) -> (-25, 17.3147)
  line L4 (-25, 17.3147) -> (-25, 17.4997)
  line L5 (-25, 5) -> (-34, 5)
  line L6 (-34, 5) -> (-34, 14)
  line L7 (-34, 14) -> (-25, 14)
  line L8 (-25, 14) -> (-25, 5)
  dimension "d147" = 9
  constraint horizontal L5
  constraint vertical L6
  constraint horizontal L7
  constraint vertical L8
  constraint coincident L2.end L3.start
  measures "d147" distance of L2.end L7.end
extrude "Extrude28" cut sketch "Sketch23" against normal blind 1.5 contours L1 L2 L3 L5 L6 L7 L8 bodies 2
sketch "Sketch24" plane through (0, 0, 26.7503) normal (0, 0, 1) x (1, 0, 0)
  line L0 (34, 17.4997) -> (25, 17.4997)
  line L1 (25, 17.4997) -> (25, 5)
  line L2 (25, 5) -> (34, 5)
  line L3 (34, 5) -> (34, 17.4997)
  line L4 (34, 5) -> (25, 5)
  line L5 (25, 5) -> (25, 14)
  line L6 (25, 14) -> (34, 14)
  line L7 (34, 14) -> (34, 5)
  dimension "d150" = 9
  constraint horizontal L4
  constraint vertical L5
  constraint horizontal L6
  constraint vertical L7
  constraint coincident L2.end L3.start
  measures "d150" distance of L2.end L6.end
extrude "Extrude29" cut sketch "Sketch24" against normal blind 1.5 contours L1 L2 L3 L4 L5 L6 L7 bodies 2
chamfer "Chamfer1" distance 1 angle 45 2 edges at (29.5, 14, 26.7503) (29.5, 14, 15.2503) on bodies 2
sketch "Sketch25" plane through (0, 17.4997, 0) normal (0, 1, 0) x (-1, 0, 0)
  line L0 (-25, 15.2503) -> (-25, 26.75)
  line L1 (-25, 26.75) -> (-25, 26.7503)
  line L2 (-25, 26.7503) -> (-34, 26.7503)
  line L3 (-34, 26.7503) -> (-34, 15.2503)
  line L4 (-34, 15.2503) -> (-25, 15.2503)
  line L5 (-34, 21.0003) -> (-29.5, 21.0003)
  circle A0 centre (-29.5, 21.0003) radius 2
  dimension "d154" = 4.5
  dimension "d155" = 4
  constraint midpoint L3 L5.start
  constraint perpendicular L3 L5
  constraint coincident L5.end A0.centre
  measures "d154" distance of L5.start L5.end
  measures "d155" diameter of A0
extrude "Extrude30" cut sketch "Sketch25" against normal blind 8 contours A0 bodies 2
sketch "Sketch26" plane through (0, 0, 26.7503) normal (0, 0, 1) x (1, 0, 0)
  line L0 (25, 15) -> (34, 15)
  line L1 (34, 15) -> (34, 17.4997)
  line L2 (34, 17.4997) -> (25, 17.4997)
  line L3 (25, 17.4997) -> (25, 15)
  circle A0 centre (29.5, 17.4997) radius 2
  dimension "d158" = 4
  constraint midpoint L2 A0.centre
  measures "d158" diameter of A0
extrude "Extrude31" cut sketch "Sketch26" against normal blind 42 contours L2 A0 picked at (30.0109, 16.7504) bodies 2
sketch "Sketch27" plane through (0, 5, 0) normal (0, 1, 0) x (-1, 0, 0)
sketch "Sketch28" plane through (0, 5, 0) normal (0, 1, 0) x (-1, 0, 0)
sketch "Sketch29" plane through (0, 0, 0) normal (0, -1, 0) x (1, 0, 0)
  arc A0 (28, 42) -> (25, 39) centre (28, 39) ccw
  line L0 (25, 39) -> (25, 23.5)
  line L1 (25, 23.5) -> (15, 23.5)
  line L2 (15, 23.5) -> (15, 18.5)
  line L3 (15, 18.5) -> (25, 18.5)
  line L4 (25, 18.5) -> (25, 3)
  arc A1 (25, 3) -> (28, 0) centre (28, 3) ccw
  line L5 (28, 0) -> (64, 0)
  arc A2 (64, 0) -> (67, 3) centre (64, 3) ccw
  line L6 (67, 3) -> (67, 39)
  arc A3 (67, 39) -> (64, 42) centre (64, 39) ccw
  line L7 (64, 42) -> (28, 42)
  circle A4 centre (46, 21) radius 12
  circle A5 centre (20, 21) radius 1.25
  circle A6 centre (30.5, 5.5) radius 1.75
  circle A7 centre (30.5, 36.5) radius 1.75
  circle A8 centre (61.5, 5.5) radius 1.75
  circle A9 centre (61.5, 36.5) radius 1.75
  circle A10 centre (30.5, 5.5) radius 3.25
  circle A11 centre (61.5, 5.5) radius 3.25
  circle A12 centre (61.5, 36.5) radius 3.25
  circle A13 centre (30.5, 36.5) radius 3.25
  dimension "d169" = 6.5
  dimension "d170" = 6.5
  dimension "d171" = 6.5
  dimension "d172" = 6.5
  constraint concentric A6 A10
  constraint concentric A8 A11
  constraint concentric A9 A12
  constraint concentric A7 A13
  measures "d169" diameter of A10
  measures "d170" diameter of A11
  measures "d171" diameter of A12
  measures "d172" diameter of A13
extrude "Extrude32" add sketch "Sketch29" against normal blind 9 contours A10 | A11 | A12 | A13 bodies 2
extrude "Extrude33" cut 2 faces at (50.1667, 17.5, 37.5) (49.1667, 17.5, 4.5) along direction (0, -1, 0) blind 12.5 on bodies 2 bodies 2
extrude "Extrude34" cut 2 faces at (44.5762, 12.5, 4.3122) (46.2821, 12.5, 37.5983) along direction (0, -1, 0) blind 7.5 on bodies 2 bodies 2
extrude "Extrude35" cut 1 faces at (33.1164, 16.4124, 15.2504) along direction (0, 0, 1) blind 17 on bodies 2 bodies 2
extrude "Extrude36" cut 2 faces at (15, 16.3867, 21.835) (15, 4.7267, 21.8333) along direction (1, 0, 0) blind 10 on bodies 2 bodies 2
extrude "Extrude37" cut 1 faces at (29.5498, 15, 25.4985) along direction (0, -1, 0) blind 10 on bodies 2 bodies 2
sketch "Sketch30" plane through (0, 5, 0) normal (0, 1, 0) x (-1, 0, 0)
  circle A0 centre (-29.5, 21.0003) radius 2
  line L0 (-25, 3) -> (-25, 39)
  arc A1 (-25, 39) -> (-28, 42) centre (-28, 39) ccw
  line L1 (-28, 42) -> (-64, 42)
  arc A2 (-64, 42) -> (-67, 39) centre (-64, 39) ccw
  line L2 (-67, 39) -> (-67, 3)
  arc A3 (-67, 3) -> (-64, 0) centre (-64, 3) ccw
  line L3 (-64, 0) -> (-28, 0)
  arc A4 (-28, 0) -> (-25, 3) centre (-28, 3) ccw
  circle A5 centre (-30.5, 5.5) radius 3.25
  circle A6 centre (-30.5, 36.5) radius 3.25
  circle A7 centre (-61.5, 5.5) radius 3.25
  circle A8 centre (-61.5, 36.5) radius 3.25
  circle A9 centre (-46, 21) radius 8.625
  circle A10 centre (-29.5, 21.0003) radius 2
  constraint concentric A0 A10
extrude "Extrude38" cut sketch "Sketch30" along normal blind 6 contours A0 A10 bodies 2
extrude "Extrude39" add 4 faces at (64.2314, 9, 5.2516) (33.2314, 9, 5.2516) (33.2314, 9, 36.2516) (64.2314, 9, 36.2516) along direction (0, 1, 0) blind 3 on bodies 2 bodies 2
sketch "Sketch31" plane through (0, 0, 42) normal (0, 0, 1) x (1, 0, 0)
  line L0 (64, 5) -> (28, 5)
  line L1 (28, 5) -> (28, 0)
  line L2 (28, 0) -> (64, 0)
  line L3 (64, 0) -> (64, 5)
  line L4 (46, 0) -> (56, 0)
  line L5 (56, 0) -> (58, 0)
  line L6 (56, 0) -> (56, 2)
  line L7 (58, 0) -> (34, 0)
  line L8 (34, 0) -> (34, 24)
  line L9 (34, 24) -> (58, 24)
  line L10 (58, 24) -> (58, 0)
  line L11 (56, 2) -> (36, 2)
  line L12 (36, 2) -> (36, 22)
  line L13 (36, 22) -> (56, 22)
  line L14 (56, 22) -> (56, 2)
  dimension "d189" = 24
  constraint midpoint L2 L4.start
  constraint coincident L2 L4.end
  constraint coincident L2 L5.end
  constraint perpendicular L0 L6
  constraint horizontal L7
  constraint vertical L8
  constraint horizontal L9
  constraint vertical L10
  constraint horizontal L11
  constraint vertical L12
  constraint horizontal L13
  constraint vertical L14
  measures "d189" distance of L5.end L9.end
extrude "Extrude40" add sketch "Sketch31" along normal blind 10 contours L0 L2 L5 L6 L7 L10 L14 | L0 L8 L9 L10 L12 L13 L14 | L0 L2 L4 L6 L7 L8 L11 L12 bodies 2
extrude "Extrude41" add 1 faces at (42, 24, 45.3333) along direction (0, 1, 0) blind 0.25 on bodies 2 bodies 2
extrude "Extrude42" cut 1 faces at (42.6667, 22, 45.3333) along direction (0, 1, 0) blind 0.25 on bodies 2 bodies 2
extrude "Extrude43" cut 1 faces at (36, 9.75, 48.6667) along direction (-1, 0, 0) blind 0.125 on bodies 2 bodies 2
extrude "Extrude44" add 1 faces at (34, 9.75, 48.6667) along direction (-1, 0, 0) blind 0.125 on bodies 2 bodies 2
extrude "Extrude45" cut 1 faces at (56, 9.75, 48.6667) along direction (1, 0, 0) blind 0.125 on bodies 2 bodies 2
extrude "Extrude46" add 1 faces at (58, 9.75, 48.6667) along direction (1, 0, 0) blind 0.125 on bodies 2 bodies 2
sketch "Sketch32" plane through (0, 0, 42) normal (0, 0, -1) x (-1, 0, 0)
  line L0 (-56.125, 5) -> (-56.125, 22.25)
  line L1 (-56.125, 22.25) -> (-35.875, 22.25)
  line L2 (-35.875, 22.25) -> (-35.875, 5)
  line L3 (-35.875, 5) -> (-33.875, 5)
  line L4 (-33.875, 5) -> (-33.875, 24.25)
  line L5 (-33.875, 24.25) -> (-58.125, 24.25)
  line L6 (-58.125, 24.25) -> (-58.125, 5)
  line L7 (-58.125, 5) -> (-56.125, 5)
  line L8 (-35.875, 5) -> (-33.875, 5)
  line L9 (-33.875, 5) -> (-33.875, 24.25)
  line L10 (-33.875, 24.25) -> (-35.875, 24.25)
  line L11 (-35.875, 24.25) -> (-35.875, 5)
  line L12 (-56.125, 5) -> (-58.125, 5)
  line L13 (-58.125, 5) -> (-58.125, 24.25)
  line L14 (-58.125, 24.25) -> (-56.125, 24.25)
  line L15 (-56.125, 24.25) -> (-56.125, 5)
  constraint horizontal L8
  constraint vertical L9
  constraint horizontal L10
  constraint vertical L11
  constraint coincident L4.end L5.start
  constraint coincident L2.end L3.start
  constraint horizontal L12
  constraint vertical L13
  constraint horizontal L14
  constraint vertical L15
  constraint coincident L5.end L6.start
  constraint coincident L0.start L7.end
extrude "Extrude47" add sketch "Sketch32" along normal blind 12 contours L0 L5 L6 L7 L12 L13 L14 L15 | L2 L3 L4 L5 L8 L9 L10 L11 bodies 2
sketch "Sketch33" plane through (35.875, 0, 0) normal (1, 0, 0) x (0, 0, -1)
  line L0 (-42, 22.25) -> (-52, 22.25)
  line L1 (-52, 22.25) -> (-52, 2)
  line L2 (-52, 2) -> (-42, 2)
  line L3 (-42, 2) -> (-42, 5)
  line L4 (-42, 5) -> (-30, 5)
  line L5 (-30, 5) -> (-30, 24.25)
  line L6 (-30, 24.25) -> (-42, 24.25)
  line L7 (-42, 24.25) -> (-42, 22.25)
  line L8 (-42, 24.25) -> (-30, 5)
  constraint coincident L6.end L7.start
  constraint coincident L4.end L5.start
extrude "Extrude48" cut sketch "Sketch33" along normal blind 22.25 and the other way blind 2 contours L5 L6 L8 bodies 2
sketch "Sketch34" plane through (0, 24.25, 0) normal (0, 1, 0) x (-1, 0, 0)
  line L0 (-35.875, 42) -> (-33.875, 42)
  line L1 (-33.875, 42) -> (-33.875, 52)
  line L2 (-33.875, 52) -> (-58.125, 52)
  line L3 (-58.125, 52) -> (-58.125, 42)
  line L4 (-58.125, 42) -> (-56.125, 42)
  line L5 (-56.125, 42) -> (-35.875, 42)
  line L6 (-46, 42) -> (-46, 47)
  circle A0 centre (-46, 47) radius 1
  dimension "d210" = 2
  constraint midpoint L5 L6.start
  constraint perpendicular L5 L6
  constraint coincident L6.end A0.centre
  measures "d210" diameter of A0
extrude "Extrude49" cut sketch "Sketch34" against normal blind 27 contours A0 bodies 2
delete_face "DeleteFace1" 1 faces at (27.8573, 1.6667, 41.9966) on bodies 2
delete_face "DeleteFace2" 1 faces at (27.8573, 1.6667, 0.0034) on bodies 2
delete_face "DeleteFace3" 1 faces at (66.0702, 1.6667, 0.8288) on bodies 2
delete_face "DeleteFace4" 1 faces at (66.1712, 1.6667, 41.0702) on bodies 2
sketch "Sketch35" plane through (0, 2, 0) normal (0, 1, 0) x (-1, 0, 0)
  circle A0 centre (-46, 47) radius 1
  line L0 (-56.125, 42) -> (-35.875, 42)
  line L1 (-35.875, 42) -> (-35.875, 52)
  line L2 (-35.875, 52) -> (-56.125, 52)
  line L3 (-56.125, 52) -> (-56.125, 42)
  line L4 (-46, 52) -> (-48.5, 52)
  line L5 (-48.5, 52) -> (-43.5, 52)
  line L6 (-43.5, 52) -> (-43.5, 42)
  line L7 (-43.5, 42) -> (-48.5, 42)
  line L8 (-48.5, 42) -> (-48.5, 52)
  dimension "d213" = 2.5
  dimension "d214" = 5
  constraint midpoint L2 L4.start
  constraint parallel L2 L4
  constraint horizontal L5
  constraint vertical L6
  constraint horizontal L7
  constraint vertical L8
  measures "d213" distance of L4.start L4.end
  measures "d214" distance of L4.end L5.end
extrude "Extrude50" add sketch "Sketch35" along normal blind 6.34 contours L0 L2 L4 L5 L6 L7 L8 bodies 2
sketch "Sketch36" plane through (0, 22.25, 0) normal (0, -1, 0) x (1, 0, 0)
  circle A0 centre (46, 47) radius 1
  line L0 (35.875, 42) -> (56.125, 42)
  line L1 (56.125, 42) -> (56.125, 52)
  line L2 (56.125, 52) -> (35.875, 52)
  line L3 (35.875, 52) -> (35.875, 42)
  line L4 (46, 52) -> (48.5, 52)
  line L5 (48.5, 52) -> (43.5, 52)
  line L6 (43.5, 52) -> (43.5, 42)
  line L7 (43.5, 42) -> (48.5, 42)
  line L8 (48.5, 42) -> (48.5, 52)
  dimension "d217" = 2.5
  dimension "d218" = 5
  constraint midpoint L2 L4.start
  constraint parallel L2 L4
  constraint horizontal L5
  constraint vertical L6
  constraint horizontal L7
  constraint vertical L8
  measures "d217" distance of L4.start L4.end
  measures "d218" distance of L4.end L5.end
extrude "Extrude51" add sketch "Sketch36" along normal blind 6.3 contours L0 L2 L4 L5 L6 L7 L8 bodies 2
extrude "Extrude52" cut 4 faces at (33.2314, 12, 5.2516) (64.2314, 12, 5.2516) (33.2314, 12, 36.2516) (64.2314, 12, 36.2516) along direction (0, -1, 0) blind 1.5 on bodies 2 bodies 2
sketch "Sketch37" plane through (0, 5, 0) normal (0, 1, 0) x (-1, 0, 0)
  line L0 (-67, 42) -> (-67, 0)
  line L1 (-67, 0) -> (-25, 0)
  line L2 (-25, 0) -> (-25, 42)
  line L3 (-25, 42) -> (-33.875, 42)
  line L4 (-33.875, 42) -> (-33.875, 30)
  line L5 (-33.875, 30) -> (-35.875, 30)
  line L6 (-35.875, 30) -> (-35.875, 42)
  line L7 (-35.875, 42) -> (-43.5, 42)
  line L8 (-43.5, 42) -> (-48.5, 42)
  line L9 (-48.5, 42) -> (-56.125, 42)
  line L10 (-56.125, 42) -> (-56.125, 30)
  line L11 (-56.125, 30) -> (-58.125, 30)
  line L12 (-58.125, 30) -> (-58.125, 42)
  line L13 (-58.125, 42) -> (-67, 42)
  circle A0 centre (-46, 21) radius 8.625
  circle A1 centre (-61.5, 36.5) radius 3.25
  circle A2 centre (-61.5, 5.5) radius 3.25
  circle A3 centre (-30.5, 36.5) radius 3.25
  circle A4 centre (-30.5, 5.5) radius 3.25
  circle A5 centre (-46, 21) radius 10
  line L14 (-46, 21) -> (-36, 21)
  line L15 (-36, 21) -> (-56, 21)
  line L16 (-56, 21) -> (-56, 42)
  line L17 (-56, 42) -> (-36, 42)
  line L18 (-36, 42) -> (-36, 21)
  dimension "d223" = 20
  dimension "d224" = 20
  constraint concentric A0 A5
  constraint coincident A0.centre A5.centre
  constraint coincident A5 L14.end
  constraint horizontal L14
  constraint horizontal L15
  constraint vertical L16
  constraint horizontal L17
  constraint vertical L18
  measures "d223" diameter of A5
  measures "d224" distance of L14.end L15.end